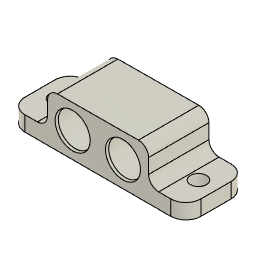
Intake+and+Outflow+Tube+Routing (Autodesk Fusion 360 design; units mm, degrees)
Autodesk Fusion 360 part; units mm, degrees
sketch "Sketch1" plane through (0, 0, 0) normal (0, 1, 0) x (1, 0, 0)
  circle A0 centre (-5, -5) radius 3.35
  circle A1 centre (5, -5) radius 3.35
  line L0 (-10, -5) -> (-10, -7.815)
  line L1 (-8.0118, -9.815) -> (8.0725, -9.9095)
  line L2 (10.0842, -7.9096) -> (10.0842, -5)
  line L3 (-17.5, 0) -> (17.5, 0)
  line L4 (17.5, 0) -> (17.5, -3)
  line L5 (-17.5, -3) -> (-17.5, 0)
  line L6 (-12, -3) -> (-17.5, -3)
  line L7 (17.5, -3) -> (12.0842, -3)
  arc A2 (-10, -7.815) -> (-8.0118, -9.815) centre (-8, -7.815) ccw
  arc A3 (-10, -5) -> (-12, -3) centre (-12, -5) ccw
  arc A4 (8.0725, -9.9095) -> (10.0842, -7.9096) centre (8.0842, -7.9096) ccw
  arc A5 (12.0842, -3) -> (10.0842, -5) centre (12.0842, -5) ccw
  point P0 (0, -5)
  dimension "d1" = 6.7
  dimension "d2" = 35
  dimension "d12" = 3
  dimension "d13" = 2
  constraint equal A0 A1
  constraint parallel L0 L2
  constraint horizontal L3
  constraint vertical L4
  constraint horizontal L7
  constraint vertical L5
  constraint midpoint origin L3
  constraint collinear L6 L7
  constraint tangent L0 A2
  constraint tangent L1 A2
  constraint tangent L6 A3
  constraint tangent L0 A3
  constraint equal A2 A3
  constraint tangent L1 A4
  constraint tangent L2 A4
  constraint equal A2 A4
  constraint tangent L7 A5
  constraint tangent L2 A5
  constraint equal A2 A5
  measures "d1" diameter of A0
  measures "d2" distance of L3.start L3.end
  measures "d12" distance of L3 L6
  measures "d13" radius of A3
extrude "Extrude1" add sketch "Sketch1" along normal blind 12
sketch "Sketch2" plane through (0, 0, 0) normal (0, 0, -1) x (1, 0, 0)
  line L0 (17.5, 0) -> (-17.5, 0)
  line L1 (-17.5, 0) -> (-17.5, -12)
  line L2 (-17.5, -12) -> (17.5, -12)
  line L3 (17.5, -12) -> (17.5, 0)
  circle A0 centre (-14, -6) radius 1.6
  circle A1 centre (14, -6) radius 1.6
  dimension "d6" = 3.2
  dimension "d7" = 3.2
  measures "d6" diameter of A0
  measures "d7" diameter of A1
extrude "Extrude2" cut sketch "Sketch2" against normal blind 5 contours A0 | A1
fillet "Fillet1" radius 3 4 edges at (17.5, 0, 1.5) (17.5, 12, 1.5) (-17.5, 0, 1.5) (-17.5, 12, 1.5)
chamfer "Chamfer1" distance 0.5 angle 15 2 edges at (-8.1233, 0, 3.7886) (1.8767, 0, 3.7886) measured on face at (-1.6542, 8, 5.167) measured on face at (8.3458, 8, 5.167)
chamfer "Chamfer1" distance 0.5 angle 15 2 edges at (1.8767, 12, 3.7886) (-8.1233, 12, 3.7886) measured on face at (8.3458, 8, 5.167) measured on face at (-1.6542, 8, 5.167)
